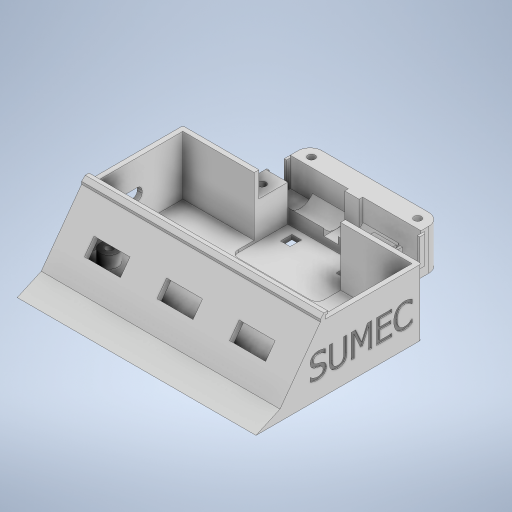
# Autodesk Inventor part: Sumec_telo_V4.1
Saved by Autodesk Inventor 2023 (Build 270158000, 158)
## iProperties
Created: 2023-03-18
Part Number: Sumec_telo_V4.1
Material: Všeobecné
Document SubType Name: Modeling
Designer: jaryj
Density: 1 g/cm^3
Appearance: Výchozí
Author: jaryj
Autodesk Inventor part; units mm, degrees
ref_plane "YZ Plane" through (0, 0, 0) normal (1, 0, 0) x (0, 1, 0)
ref_plane "XZ Plane" through (0, 0, 0) normal (0, 1, 0) x (-1, 0, 0)
ref_plane "XY Plane" through (0, 0, 0) normal (0, 0, 1) x (1, 0, 0)
sketch "Náčrt1" plane through (0, 0, 0) normal (0, 1, 0) x (-1, 0, 0)
  line L0 (0, 0) -> (49.75, 0)
  line L1 (49.75, 0) -> (49.75, -69)
  line L2 (49.75, -69) -> (18, -69)
  line L3 (18, -69) -> (18, -81)
  line L4 (18, -81) -> (27.25, -81)
  line L5 (27.25, -81) -> (27.25, -69)
  line L6 (27.25, -81) -> (27.25, -91.25)
  line L7 (27.25, -91.25) -> (27.25, -99.5)
  line L8 (27.25, -99.5) -> (0, -99.5)
  line L9 (0, -99.5) -> (0, -91.25)
  line L10 (0, -91.25) -> (27.25, -91.25)
  line L11 (0, -91.25) -> (0, -81)
  line L12 (0, -81) -> (18, -81)
  line L13 (0, -81) -> (0, 0)
  line L14 (18, -69) -> (18, -57.25)
  line L15 (18, -57.25) -> (0, -57.25)
  line L16 (47.75, -30) -> (47.75, -67)
  line L17 (47.75, -67) -> (18, -67)
  line L18 (0, -30) -> (47.75, -30)
  dimension "d0" = 49.75
  dimension "d1" = 69
  dimension "d2" = 12
  dimension "d3" = 10.25
  dimension "d4" = 8.25
  dimension "d5" = 27.25
  dimension "d6" = 18
  dimension "d9" = 2
  dimension "d13" = 30
  dimension "d18" = 2
  dimension "d190" = 9.75
  constraints: 38 end point, 12 perpendicular, 7 point on line, 1 horizontal, 1 vertical
  measures "d0" distance of L0.start L0.end
  measures "d1" distance of L0.end L1.end
  measures "d2" distance of L4.end L5.end
  measures "d3" distance of L4.end L6.end
  measures "d4" distance of L6.end L7.end
  measures "d5" distance of L7.end L8.end
  measures "d6" distance of L3.end L11.end
  measures "d9" distance between parallel lines of L17 L2
  measures "d13" distance between parallel lines of L0 L18
  measures "d18" distance between parallel lines of L1 L16
  measures "d190" distance between parallel lines of L17 L15
extrude "Vysunutí1" add sketch "Náčrt1" along normal blind 3 contours L18 L16 L17 L14 L15 L13
extrude "Vysunutí2" add sketch "Náčrt1" along normal blind 1.888 contours L15 L14 L3 L12 L13
extrude "Vysunutí3" add sketch "Náčrt1" along normal blind 27.5 contours L0 L1 L2 L14 L17 L16 L18 L13
extrude "Vysunutí4" add sketch "Náčrt1" along normal blind 17 contours L5 L4 L3 L2 | L10 L7 L8 L9
extrude "Vysunutí15" add sketch "Náčrt1" along normal blind 5 contours L12 L4 L6 L10 L11
sketch "Náčrt2" plane through (-49.75, 0, -69) normal (-1, 0, 0) x (0, 0, 1)
  line L0 (69, 0) -> (69, 27.5) projected
  line L1 (69, 0) -> (59, 4.5)
  line L2 (0, 0) -> (69, 0) projected
  line L3 (42.1707, 27.5) -> (59, 4.5)
  line L4 (69, 27.5) -> (0, 27.5) projected
  line L5 (69, 0) -> (69, 27.5) projected
  line L6 (69, 0) -> (69, 27.5)
  line L7 (69, 27.5) -> (42.1707, 27.5)
  point P0 (39, 27.5)
  point P1 (45.8293, 22.5)
  dimension "d24" = 4.5
  dimension "d25" = 10
  dimension "d235" = 53.807
  constraints: 8 end point, 1 collinear, 1 perpendicular, 1 point on line
  measures "d24" distance from line of L2 L1.end
  measures "d25" horizontal distance of L0.start L1.end
  measures "d235" angle of L2 L3
extrude "Vysunutí6" cut sketch "Náčrt2" against normal up to surface (49.75 mm away)
sketch "Náčrt3" plane through (0, 3, -30) normal (0, 0, -1) x (-1, 0, 0)
  line L0 (22.75, 15.167) -> (37.75, 15.167)
  line L1 (37.75, 15.167) -> (37.75, 0)
  line L2 (37.75, 0) -> (22.75, 0)
  line L3 (22.75, 0) -> (22.75, 15.167)
  line L4 (0, 15.167) -> (7.5, 15.167)
  line L5 (7.5, 15.167) -> (7.5, 0)
  line L6 (7.5, 0) -> (0, 0)
  line L7 (0, 0) -> (0, 15.167)
  line L8 (49.75, -3) -> (0, -3) projected
  dimension "d30" = 15
  dimension "d31" = 7.5
  dimension "d32" = 15.167
  dimension "d33" = 3
  dimension "d34" = 15.25
  constraints: 16 end point, 4 perpendicular, 4 point on line, 1 horizontal, 1 vertical alignment
  measures "d30" distance of L0.start L0.end
  measures "d31" distance of L4.start L4.end
  measures "d32" distance of L0.end L1.end
  measures "d33" distance between parallel lines of L8 L6
  measures "d34" distance between parallel lines of L3 L5
extrude "Vysunutí7" cut sketch "Náčrt3" against normal blind 14
sketch "Náčrt7" plane through (-47.75, 3, -67) normal (1, 0, 0) x (0, 0, -1)
  line L0 (-37, 0) -> (-50, 0)
  line L1 (-37, 0) -> (-51, 0) projected
  line L2 (-50, 0) -> (-50, 6.833)
  line L3 (-40.1707, 24.5) -> (2, 24.5) projected
  line L4 (2, -3) -> (-67, -3) projected
  line L5 (-40.1707, 24.5) -> (-46.9998, 15.167) projected
  line L6 (-37, 15.167) -> (-37, 24.5) projected
  line L7 (-37, 24.5) -> (-37, 0)
  line L8 (-37, 24.5) -> (-40.1707, 24.5) projected
  line L9 (-37.073, 24.5) -> (-37, 24.5)
  line L10 (-50, 6.833) -> (-37.073, 24.5)
  point P0 (-37, 15.167)
  dimension "d45" = 13
  dimension "d261" = 2.5
  constraints: 10 end point, 3 collinear, 2 perpendicular, 1 point on line
  measures "d45" distance of L0.start L0.end
  measures "d261" distance between parallel lines of L10 L5
extrude "Vysunutí9" cut sketch "Náčrt7" along normal through all
sketch "Náčrt13" plane through (0, 17, 0) normal (0, 1, 0) x (1, 0, 0)
  line L0 (-27.25, 81) -> (-18, 81) projected
  line L1 (-27.25, 69) -> (-27.25, 81) projected
  point P0 (0, 0)
  point P1 (-22.625, 75)
  dimension "d84" = 6
  dimension "d85" = 4.625
  measures "d84" distance from line of L0 point (-22.625, 75)
  measures "d85" distance from line of L1 point (-22.625, 75)
hole "Díra2" at (-22.625, 17, -75) direction (0, -1, 0) diameter 3 depth 6
sketch "Náčrt14" plane through (0, 17, 0) normal (0, 1, 0) x (1, 0, 0)
  line L0 (-27.25, 91.25) -> (-27.25, 99.5) projected
  line L1 (-27.25, 99.5) -> (0, 99.5) projected
  point P0 (0, 0)
  point P1 (-22.125, 95)
  dimension "d93" = 5.125
  dimension "d101" = 4.5
  measures "d93" distance from line of L0 point (-22.125, 95)
  measures "d101" distance from line of L1 point (-22.125, 95)
hole "Díra3" at (-22.125, 17, -95) direction (0, -1, 0) diameter 3 depth 6
fillet "Zaoblení1" radius 3 1 edges at (-18, 2.444, -57.25)
fillet "Zaoblení2" radius 1 1 edges at (-49.75, 13.75, -69)
fillet "Zaoblení3" radius 5 1 edges at (-27.25, 8.5, -99.5)
sketch "Náčrt24" plane through (-18, 3, -67) normal (1, 0, 0) x (0, 0, -1)
  line L0 (24.25, 2) -> (24.25, 14) projected
  line L1 (14, 2) -> (24.25, 2) projected
  line L2 (14, 2) -> (14, 14) projected
  line L3 (24.25, 2) -> (14, 2) projected
  line L4 (24.25, 4.88) -> (24.25, 2)
  line L5 (24.25, 2) -> (14, 2)
  line L6 (14, 2) -> (14, 4.88)
  arc A0 (14, 4.88) -> (24.25, 4.88) centre (19.125, 8) ccw
  point P0 (-67, -3)
  point P1 (19.125, 2)
  dimension "d200" = 6
  constraints: 6 end point, 2 perpendicular, 2 point on circle, 2 point on line, 1 centre point, 1 horizontal alignment, 1 tangent
  measures "d200" radius of A0
extrude "Vysunutí22" add sketch "Náčrt24" along normal blind 15
sketch "Náčrt21" plane through (-27.25, 0, -69) normal (-1, 0, 0) x (0, 0, 1)
  line L0 (-20.75, 16) -> (-23.75, 16)
  line L1 (-30.5, 17) -> (-22.25, 17) projected
  line L2 (-23.75, 3.5) -> (-10.5, 3.5)
  line L3 (-10.5, 3.5) -> (-10.5, 16)
  line L4 (-10.5, 16) -> (-13.5, 16)
  line L5 (-13.5, 16) -> (-13.5, 6.5)
  line L6 (-13.5, 6.5) -> (-20.75, 6.5)
  line L7 (-20.75, 6.5) -> (-20.75, 16)
  line L8 (-23.75, 16) -> (-23.75, 3.5)
  line L9 (-22.25, 5) -> (-22.25, 17) projected
  line L10 (-12, 5) -> (-22.25, 5) projected
  line L11 (-12, 5) -> (-12, 17) projected
  line L12 (0, 17) -> (-12, 17) projected
  point P0 (69, 0)
  dimension "d172" = 1.5
  dimension "d173" = 1.5
  dimension "d174" = 1.5
  dimension "d175" = 1.5
  dimension "d176" = 1.5
  dimension "d177" = 1.5
  dimension "d180" = 1
  constraints: 12 end point, 3 perpendicular, 1 horizontal, 1 parallel, 1 vertical, 8 other
  measures "d172" distance between parallel lines of L7 L9
  measures "d173" distance between parallel lines of L6 L10
  measures "d174" distance between parallel lines of L5 L11
  measures "d175" distance between parallel lines of L11 L3
  measures "d176" distance between parallel lines of L2 L10
  measures "d177" distance between parallel lines of L8 L9
extrude "Vysunutí19" add sketch "Náčrt21" along normal blind 1
chamfer "Zkosení1" distance 1 angle 45 3 edges at (-28.25, 9.75, -92.75) (-28.25, 3.5, -86.125) (-28.25, 9.75, -79.5)
mirror "Zrcadlit1" about plane through (0, 0, -99.5) normal (1, 0, 0)
sketch "Náčrt30" plane through (-49.75, 0, -68) normal (-1, 0, 0) x (0, 0, 1)
  line L0 (58, 4.5) -> (41.1707, 27.5) projected
  line L1 (41.1707, 27.5) -> (41.1707, 30)
  line L2 (41.1707, 30) -> (38.073, 30)
  line L3 (38.073, 30) -> (38.073, 29)
  line L4 (38.073, 29) -> (39.073, 29)
  line L5 (39.073, 29) -> (39.073, 27.5)
  line L6 (41.1707, 27.5) -> (0, 27.5) projected
  line L7 (39.073, 27.5) -> (41.1707, 27.5)
  line L8 (38.073, 27.5) -> (51, 9.833) projected
  point P0 (68, 0)
  point P1 (39.073, 27.5)
  dimension "d236" = 1.5
  dimension "d237" = 1
  dimension "d263" = 1
  constraints: 12 end point, 4 perpendicular, 1 collinear, 1 horizontal, 1 vertical alignment
  measures "d236" distance of L4.end L5.end
  measures "d237" distance of L3.end L4.end
  measures "d263" distance of L2.end L3.end
sketch "Náčrt16" plane through (0, 1.888, 0) normal (0, 1, 0) x (1, 0, 0)
  line L0 (-9.4, 73.375) -> (-13.4, 73.375)
  line L1 (-13.4, 73.375) -> (-13.4, 78.125)
  line L2 (-13.4, 78.125) -> (-9.4, 78.125)
  line L3 (-9.4, 78.125) -> (-9.4, 73.375)
  line L4 (-18, 81) -> (-18, 69) projected
  line L5 (13.75, 73.375) -> (9.75, 73.375)
  line L6 (9.75, 73.375) -> (9.75, 78.125)
  line L7 (9.75, 78.125) -> (13.75, 78.125)
  line L8 (13.75, 78.125) -> (13.75, 73.375)
  line L9 (18, 81) -> (18, 69) projected
  line L10 (-18, 81) -> (18, 81) projected
  point P0 (0, 0)
  dimension "d128" = 4
  dimension "d129" = 4.75
  dimension "d130" = 4.6
  dimension "d134" = 4.25
  dimension "d192" = 2.875
  constraints: 16 end point, 4 parallel, 2 equal length, 2 perpendicular, 1 horizontal, 1 horizontal alignment
  measures "d128" distance of L0.start L0.end
  measures "d129" distance of L2.end L0.start
  measures "d130" distance between parallel lines of L4 L1
  measures "d134" distance between parallel lines of L9 L8
  measures "d192" distance between parallel lines of L10 L2
extrude "Vysunutí16" cut sketch "Náčrt16" against normal through all
sketch "Náčrt17" plane through (0, 3, 0) normal (0, 1, 0) x (1, 0, 0)
  line L0 (-47.75, 17) -> (-37.75, 17) projected
  line L1 (-47.75, 17) -> (-47.75, 67) projected
  line L2 (47.75, 17) -> (37.75, 17) projected
  line L3 (47.75, 17) -> (47.75, 67) projected
  line L4 (-39.4, 19.625) -> (-43.4, 19.625)
  line L5 (-43.4, 19.625) -> (-43.4, 24.375)
  line L6 (-43.4, 24.375) -> (-39.4, 24.375)
  line L7 (-39.4, 24.375) -> (-39.4, 19.625)
  line L8 (42.75, 19.625) -> (38.75, 19.625)
  line L9 (38.75, 19.625) -> (38.75, 24.375)
  line L10 (38.75, 24.375) -> (42.75, 24.375)
  line L11 (42.75, 24.375) -> (42.75, 19.625)
  point P0 (0, 0)
  point P1 (-48, 67)
  point P2 (48, 67)
  point P3 (-41.4, 19.625)
  point P4 (40.75, 19.625)
  point P5 (-47.75, 67)
  dimension "d137" = 4
  dimension "d138" = 4.75
  dimension "d139" = 4.35
  dimension "d143" = 2.625
  dimension "d144" = 5
  dimension "d146" = 2.625
  constraints: 16 end point, 4 parallel, 2 equal length, 2 horizontal, 2 midpoint, 2 perpendicular, 2 other
  measures "d137" distance of L4.start L4.end
  measures "d138" distance of L6.end L4.start
  measures "d143" distance between parallel lines of L0 L4
  measures "d146" distance from line of L2 point (40.75, 19.625)
extrude "Vysunutí17" cut sketch "Náčrt17" against normal through all
sketch "Náčrt18" plane through (0, 3, 0) normal (0, 1, 0) x (1, 0, 0)
  circle A0 centre (39.25, 59) radius 3.75
  circle A1 centre (-40.5, 29) radius 3.75
  line L0 (18, 67) -> (47.75, 67) projected
  line L1 (-47.75, 17) -> (-37.75, 17) projected
  line L2 (-47.75, 17) -> (-47.75, 67) projected
  line L3 (47.75, 17) -> (47.75, 67) projected
  point P0 (0, 0)
  point P1 (42.5, 67)
  point P2 (-48, 67)
  point P3 (-47.75, 67)
  dimension "d149" = 7.5
  dimension "d150" = 8
  dimension "d152" = 12
  dimension "d153" = 7.25
  dimension "d262" = 8.5
  constraints: 2 centre point, 1 equal radius, 1 other
  measures "d149" diameter of A0
  measures "d150" distance from line of A0.centre L0
  measures "d152" distance from line of L1 A1.centre
  measures "d262" distance from line of L3 A0.centre
extrude "Vysunutí18" add sketch "Náčrt18" along normal blind 5
sketch "Náčrt19" plane through (39.25, 8, -59) normal (0, 1, 0) x (1, 0, 0)
  circle A0 centre (0, 0) radius 3.75 projected
  point P0 (-39.25, -59)
  constraints: 1 coincident
hole "Díra4" at (39.25, 8, -59) direction (0, -1, 0) diameter 3 depth 6
sketch "Náčrt20" plane through (-40.5, 8, -29) normal (0, 1, 0) x (1, 0, 0)
  circle A0 centre (0, 0) radius 3.75 projected
  point P0 (40.5, -29)
  point P1 (-3.6436, 0.8871)
  point P2 (3.75, 0)
  constraints: 1 coincident
hole "Díra5" at (-40.5, 8, -29) direction (0, -1, 0) diameter 3 depth 6
sketch "Náčrt25" plane through (-18, 7.88, -91.25) normal (0, 0, 1) x (1, 0, 0)
  line L0 (40.25, 9.12) -> (-4.25, 9.12) projected
  line L1 (15, 9.12) -> (21, 9.12)
  line L2 (21, 9.12) -> (21, -2.88)
  line L3 (21, -2.88) -> (15, -2.88)
  line L4 (15, -2.88) -> (15, 9.12)
  line L5 (15, -2.88) -> (15, 0) projected
  line L6 (21, -2.88) -> (21, 0) projected
  point P0 (18, -7.88)
  dimension "d203" = 12
  dimension "d204" = 6
  constraints: 8 end point, 2 parallel, 1 coincident, 1 horizontal, 1 perpendicular, 1 point on line
  measures "d203" distance of L3.end L1.start
  measures "d204" distance between parallel lines of L2 L4
extrude "Vysunutí23" add sketch "Náčrt25" along normal blind 1.5
sketch "Náčrt26" plane through (-49.75, 0, -68) normal (-1, 0, 0) x (0, 0, 1)
  line L0 (20, 11.7) -> (27, 11.7)
  line L1 (27, 16.7) -> (20, 16.7)
  line L2 (18, 14.7) -> (18, 13.7)
  line L3 (29, 14.7) -> (29, 13.7)
  line L4 (0, 0) -> (68, 0) projected
  line L5 (0, 0) -> (0, 27.5) projected
  arc A0 (20, 16.7) -> (18, 14.7) centre (20, 14.7) ccw
  arc A1 (18, 13.7) -> (20, 11.7) centre (20, 13.7) ccw
  arc A2 (29, 14.7) -> (27, 16.7) centre (27, 14.7) ccw
  arc A3 (27, 11.7) -> (29, 13.7) centre (27, 13.7) ccw
  dimension "d207" = 11.7
  dimension "d208" = 5
  dimension "d209" = 11
  dimension "d210" = 18
  dimension "d211" = 2
  constraints: 8 end point, 8 point on circle, 8 tangent, 4 centre point, 3 equal radius, 1 horizontal, 1 parallel, 1 vertical
  measures "d207" distance between parallel lines of L4 L0
  measures "d208" distance between parallel lines of L0 L1
  measures "d209" distance between parallel lines of L3 L2
  measures "d210" distance between parallel lines of L5 L2
  measures "d211" radius of A0
extrude "Vysunutí24" cut sketch "Náčrt26" against normal up to surface (2 mm away)
sketch "Náčrt28" plane through (49.75, 0, 0) normal (1, 0, 0) x (0, 0, -1)
  line L0 (22, 17.5) -> (66, 17.5) construction
  line L1 (66, 17.5) -> (66, 7) construction
  line L2 (66, 7) -> (22, 7) construction
  line L3 (22, 7) -> (22, 17.5) construction
  line L4 (26.8293, 27.5) -> (68, 27.5) projected
  line L5 (68, 0) -> (68, 27.5) projected
  line L6 (69, 27.5) -> (69, 0) projected
  spline S0 degree 2 poles (25.8006, 7.1434) (24.7147, 7.1434) (23.1912, 7.5972) (22.5186, 7.9214) knots 0 0 0 1 2 2 2
  line L7 (22.5186, 7.9214) -> (22.5186, 9.5908)
  line L8 (22.5186, 9.5908) -> (22.6159, 9.5908)
  spline S1 degree 2 poles (22.6159, 9.5908) (23.2723, 8.9749) (24.9335, 8.2942) (25.7034, 8.2942) knots 0 0 0 1 2 2 2
  spline S2 degree 2 poles (25.7034, 8.2942) (26.8055, 8.2942) (27.9319, 9.2099) (27.9319, 9.9635) knots 0 0 0 1 2 2 2
  spline S3 degree 2 poles (27.9319, 9.9635) (27.9319, 10.5632) (27.3404, 11.3088) (26.7002, 11.4951) knots 0 0 0 1 2 2 2
  spline S4 degree 2 poles (26.7002, 11.4951) (26.2382, 11.6248) (25.4684, 11.8031) (24.893, 11.9489) knots 0 0 0 1 2 2 2
  spline S5 degree 2 poles (24.893, 11.9489) (24.3744, 12.0867) (23.5559, 12.5) (23.2399, 12.8323) knots 0 0 0 1 2 2 2
  spline S6 degree 2 poles (23.2399, 12.8323) (22.9319, 13.1645) (22.5916, 14.0559) (22.5916, 14.6394) knots 0 0 0 1 2 2 2
  spline S7 degree 2 poles (22.5916, 14.6394) (22.5916, 15.8549) (24.4878, 17.5) (25.9546, 17.5) knots 0 0 0 1 2 2 2
  spline S8 degree 2 poles (25.9546, 17.5) (26.7974, 17.5) (28.2885, 17.1677) (28.9287, 16.8517) knots 0 0 0 1 2 2 2
  line L9 (28.9287, 16.8517) -> (28.9287, 15.2634)
  line L10 (28.9287, 15.2634) -> (28.8314, 15.2634)
  spline S9 degree 2 poles (28.8314, 15.2634) (28.3533, 15.701) (26.8622, 16.3493) (26.0438, 16.3493) knots 0 0 0 1 2 2 2
  spline S10 degree 2 poles (26.0438, 16.3493) (25.1199, 16.3493) (23.9773, 15.4822) (23.9773, 14.7771) knots 0 0 0 1 2 2 2
  spline S11 degree 2 poles (23.9773, 14.7771) (23.9773, 14.1451) (24.6499, 13.3914) (25.282, 13.2212) knots 0 0 0 1 2 2 2
  spline S12 degree 2 poles (25.282, 13.2212) (25.7034, 13.1078) (26.9271, 12.816) (27.3323, 12.6945) knots 0 0 0 1 2 2 2
  spline S13 degree 2 poles (27.3323, 12.6945) (28.3614, 12.3784) (29.3177, 11.1062) (29.3177, 10.1742) knots 0 0 0 1 2 2 2
  spline S14 degree 2 poles (29.3177, 10.1742) (29.3177, 9.5827) (28.8395, 8.4481) (28.41, 8.0511) knots 0 0 0 1 2 2 2
  spline S15 degree 2 poles (28.41, 8.0511) (27.9319, 7.6135) (26.7164, 7.1434) (25.8006, 7.1434) knots 0 0 0 1 2 2 2
  spline S16 degree 2 poles (34.1637, 7.111) (33.2804, 7.111) (31.9676, 7.5729) (31.5057, 8.0348) knots 0 0 0 1 2 2 2
  spline S17 degree 2 poles (31.5057, 8.0348) (30.9789, 8.5535) (30.5494, 10.0122) (30.5494, 11.0818) knots 0 0 0 1 2 2 2
  line L11 (30.5494, 11.0818) -> (30.5494, 17.3217)
  line L12 (30.5494, 17.3217) -> (31.8784, 17.3217)
  line L13 (31.8784, 17.3217) -> (31.8784, 11.0818)
  spline S18 degree 2 poles (31.8784, 11.0818) (31.8784, 10.3849) (32.0567, 9.4449) (32.3079, 9.064) knots 0 0 0 1 2 2 2
  spline S19 degree 2 poles (32.3079, 9.064) (32.5754, 8.6588) (33.4992, 8.2455) (34.1637, 8.2455) knots 0 0 0 1 2 2 2
  spline S20 degree 2 poles (34.1637, 8.2455) (34.7877, 8.2455) (35.7601, 8.6588) (36.0276, 9.064) knots 0 0 0 1 2 2 2
  spline S21 degree 2 poles (36.0276, 9.064) (36.2788, 9.4449) (36.4571, 10.3768) (36.4571, 11.0494) knots 0 0 0 1 2 2 2
  line L14 (36.4571, 11.0494) -> (36.4571, 17.3217)
  line L15 (36.4571, 17.3217) -> (37.7861, 17.3217)
  line L16 (37.7861, 17.3217) -> (37.7861, 11.0818)
  spline S22 degree 2 poles (37.7861, 11.0818) (37.7861, 10.0365) (37.3647, 8.5454) (36.8298, 8.0348) knots 0 0 0 1 2 2 2
  spline S23 degree 2 poles (36.8298, 8.0348) (36.3517, 7.5648) (35.0875, 7.111) (34.1637, 7.111) knots 0 0 0 1 2 2 2
  line L17 (48.2642, 7.3217) -> (46.9352, 7.3217)
  line L18 (46.9352, 7.3217) -> (46.9352, 15.936)
  line L19 (46.9352, 15.936) -> (44.3258, 10.077)
  line L20 (44.3258, 10.077) -> (43.5154, 10.077)
  line L21 (43.5154, 10.077) -> (40.9303, 15.936)
  line L22 (40.9303, 15.936) -> (40.9303, 7.3217)
  line L23 (40.9303, 7.3217) -> (39.6904, 7.3217)
  line L24 (39.6904, 7.3217) -> (39.6904, 17.3217)
  line L25 (39.6904, 17.3217) -> (41.5057, 17.3217)
  line L26 (41.5057, 17.3217) -> (44.0016, 11.7545)
  line L27 (44.0016, 11.7545) -> (46.4165, 17.3217)
  line L28 (46.4165, 17.3217) -> (48.2642, 17.3217)
  line L29 (48.2642, 17.3217) -> (48.2642, 7.3217)
  line L30 (50.2901, 7.3217) -> (50.2901, 17.3217)
  line L31 (50.2901, 17.3217) -> (56.5462, 17.3217)
  line L32 (56.5462, 17.3217) -> (56.5462, 16.1386)
  line L33 (56.5462, 16.1386) -> (51.6191, 16.1386)
  line L34 (51.6191, 16.1386) -> (51.6191, 13.3995)
  line L35 (51.6191, 13.3995) -> (56.2139, 13.3995)
  line L36 (56.2139, 13.3995) -> (56.2139, 12.2164)
  line L37 (56.2139, 12.2164) -> (51.6191, 12.2164)
  line L38 (51.6191, 12.2164) -> (51.6191, 8.5049)
  line L39 (51.6191, 8.5049) -> (56.5462, 8.5049)
  line L40 (56.5462, 8.5049) -> (56.5462, 7.3217)
  line L41 (56.5462, 7.3217) -> (50.2901, 7.3217)
  spline S24 degree 2 poles (61.9109, 7.1434) (60.9384, 7.1434) (59.2934, 7.7998) (58.6937, 8.4562) knots 0 0 0 1 2 2 2
  spline S25 degree 2 poles (58.6937, 8.4562) (58.094, 9.1045) (57.4376, 11.0494) (57.4376, 12.3136) knots 0 0 0 1 2 2 2
  spline S26 degree 2 poles (57.4376, 12.3136) (57.4376, 13.5697) (58.0778, 15.4335) (58.6856, 16.1224) knots 0 0 0 1 2 2 2
  spline S27 degree 2 poles (58.6856, 16.1224) (59.2853, 16.795) (60.9222, 17.5) (61.9352, 17.5) knots 0 0 0 1 2 2 2
  spline S28 degree 2 poles (61.9352, 17.5) (62.4376, 17.5) (63.3209, 17.3541) (63.6937, 17.2407) knots 0 0 0 1 2 2 2
  spline S29 degree 2 poles (63.6937, 17.2407) (64.0178, 17.1353) (64.6904, 16.8355) (65.0227, 16.6572) knots 0 0 0 1 2 2 2
  line L42 (65.0227, 16.6572) -> (65.0227, 15.0527)
  line L43 (65.0227, 15.0527) -> (64.9173, 15.0527)
  spline S30 degree 2 poles (64.9173, 15.0527) (64.7391, 15.2147) (64.188, 15.6686) (63.7909, 15.8874) knots 0 0 0 1 2 2 2
  spline S31 degree 2 poles (63.7909, 15.8874) (63.41, 16.0981) (62.5105, 16.3655) (61.9271, 16.3655) knots 0 0 0 1 2 2 2
  spline S32 degree 2 poles (61.9271, 16.3655) (61.2869, 16.3655) (60.1442, 15.8387) (59.7147, 15.3363) knots 0 0 0 1 2 2 2
  spline S33 degree 2 poles (59.7147, 15.3363) (59.2934, 14.8258) (58.8233, 13.278) (58.8233, 12.3136) knots 0 0 0 1 2 2 2
  spline S34 degree 2 poles (58.8233, 12.3136) (58.8233, 11.2844) (59.3177, 9.8015) (59.7472, 9.2909) knots 0 0 0 1 2 2 2
  spline S35 degree 2 poles (59.7472, 9.2909) (60.1686, 8.7966) (61.295, 8.2942) (61.9271, 8.2942) knots 0 0 0 1 2 2 2
  spline S36 degree 2 poles (61.9271, 8.2942) (62.5024, 8.2942) (63.483, 8.5778) (63.8639, 8.7885) knots 0 0 0 1 2 2 2
  spline S37 degree 2 poles (63.8639, 8.7885) (64.2285, 8.9992) (64.7715, 9.4368) (64.9254, 9.5908) knots 0 0 0 1 2 2 2
  line L44 (64.9254, 9.5908) -> (65.0227, 9.5908)
  line L45 (65.0227, 9.5908) -> (65.0227, 8.0024)
  spline S38 degree 2 poles (65.0227, 8.0024) (64.6904, 7.8485) (64.107, 7.5648) (63.6937, 7.4352) knots 0 0 0 1 2 2 2
  spline S39 degree 2 poles (63.6937, 7.4352) (63.2561, 7.2893) (62.5105, 7.1434) (61.9109, 7.1434) knots 0 0 0 1 2 2 2
  point P0 (0, 0)
  point P1 (25, 22.5)
  point P2 (0, 27.5)
  dimension "d229" = 10
  dimension "d231" = 44
  dimension "d232" = 10.5
  dimension "d264" = 3
  constraints: 3 other
  measures "d231" distance of L0.start L0.end
  measures "d232" distance of L2.end L0.start
  measures "d264" distance between parallel lines of L6 L1
extrude "Vysunutí26" cut sketch "Náčrt28" against normal blind 0.4
sketch "Náčrt29" plane through (-49.75, 0, -68) normal (-1, 0, 0) x (0, 0, 1)
  line L0 (2, 17.5) -> (46, 17.5) construction
  line L1 (46, 17.5) -> (46, 7) construction
  line L2 (46, 7) -> (2, 7) construction
  line L3 (2, 7) -> (2, 17.5) construction
  line L4 (41.1707, 27.5) -> (0, 27.5) projected
  line L5 (-1, 27.5) -> (-1, 0) projected
  spline S0 degree 2 poles (5.8006, 7.1434) (4.7147, 7.1434) (3.1912, 7.5972) (2.5186, 7.9214) knots 0 0 0 1 2 2 2
  line L6 (2.5186, 7.9214) -> (2.5186, 9.5908)
  line L7 (2.5186, 9.5908) -> (2.6159, 9.5908)
  spline S1 degree 2 poles (2.6159, 9.5908) (3.2723, 8.9749) (4.9335, 8.2942) (5.7034, 8.2942) knots 0 0 0 1 2 2 2
  spline S2 degree 2 poles (5.7034, 8.2942) (6.8055, 8.2942) (7.9319, 9.2099) (7.9319, 9.9635) knots 0 0 0 1 2 2 2
  spline S3 degree 2 poles (7.9319, 9.9635) (7.9319, 10.5632) (7.3404, 11.3088) (6.7002, 11.4951) knots 0 0 0 1 2 2 2
  spline S4 degree 2 poles (6.7002, 11.4951) (6.2382, 11.6248) (5.4684, 11.8031) (4.893, 11.9489) knots 0 0 0 1 2 2 2
  spline S5 degree 2 poles (4.893, 11.9489) (4.3744, 12.0867) (3.5559, 12.5) (3.2399, 12.8323) knots 0 0 0 1 2 2 2
  spline S6 degree 2 poles (3.2399, 12.8323) (2.9319, 13.1645) (2.5916, 14.0559) (2.5916, 14.6394) knots 0 0 0 1 2 2 2
  spline S7 degree 2 poles (2.5916, 14.6394) (2.5916, 15.8549) (4.4878, 17.5) (5.9546, 17.5) knots 0 0 0 1 2 2 2
  spline S8 degree 2 poles (5.9546, 17.5) (6.7974, 17.5) (8.2885, 17.1677) (8.9287, 16.8517) knots 0 0 0 1 2 2 2
  line L8 (8.9287, 16.8517) -> (8.9287, 15.2634)
  line L9 (8.9287, 15.2634) -> (8.8314, 15.2634)
  spline S9 degree 2 poles (8.8314, 15.2634) (8.3533, 15.701) (6.8622, 16.3493) (6.0438, 16.3493) knots 0 0 0 1 2 2 2
  spline S10 degree 2 poles (6.0438, 16.3493) (5.1199, 16.3493) (3.9773, 15.4822) (3.9773, 14.7771) knots 0 0 0 1 2 2 2
  spline S11 degree 2 poles (3.9773, 14.7771) (3.9773, 14.1451) (4.6499, 13.3914) (5.282, 13.2212) knots 0 0 0 1 2 2 2
  spline S12 degree 2 poles (5.282, 13.2212) (5.7034, 13.1078) (6.9271, 12.816) (7.3323, 12.6945) knots 0 0 0 1 2 2 2
  spline S13 degree 2 poles (7.3323, 12.6945) (8.3614, 12.3784) (9.3177, 11.1062) (9.3177, 10.1742) knots 0 0 0 1 2 2 2
  spline S14 degree 2 poles (9.3177, 10.1742) (9.3177, 9.5827) (8.8395, 8.4481) (8.41, 8.0511) knots 0 0 0 1 2 2 2
  spline S15 degree 2 poles (8.41, 8.0511) (7.9319, 7.6135) (6.7164, 7.1434) (5.8006, 7.1434) knots 0 0 0 1 2 2 2
  spline S16 degree 2 poles (14.1637, 7.111) (13.2804, 7.111) (11.9676, 7.5729) (11.5057, 8.0348) knots 0 0 0 1 2 2 2
  spline S17 degree 2 poles (11.5057, 8.0348) (10.9789, 8.5535) (10.5494, 10.0122) (10.5494, 11.0818) knots 0 0 0 1 2 2 2
  line L10 (10.5494, 11.0818) -> (10.5494, 17.3217)
  line L11 (10.5494, 17.3217) -> (11.8784, 17.3217)
  line L12 (11.8784, 17.3217) -> (11.8784, 11.0818)
  spline S18 degree 2 poles (11.8784, 11.0818) (11.8784, 10.3849) (12.0567, 9.4449) (12.3079, 9.064) knots 0 0 0 1 2 2 2
  spline S19 degree 2 poles (12.3079, 9.064) (12.5754, 8.6588) (13.4992, 8.2455) (14.1637, 8.2455) knots 0 0 0 1 2 2 2
  spline S20 degree 2 poles (14.1637, 8.2455) (14.7877, 8.2455) (15.7601, 8.6588) (16.0276, 9.064) knots 0 0 0 1 2 2 2
  spline S21 degree 2 poles (16.0276, 9.064) (16.2788, 9.4449) (16.4571, 10.3768) (16.4571, 11.0494) knots 0 0 0 1 2 2 2
  line L13 (16.4571, 11.0494) -> (16.4571, 17.3217)
  line L14 (16.4571, 17.3217) -> (17.7861, 17.3217)
  line L15 (17.7861, 17.3217) -> (17.7861, 11.0818)
  spline S22 degree 2 poles (17.7861, 11.0818) (17.7861, 10.0365) (17.3647, 8.5454) (16.8298, 8.0348) knots 0 0 0 1 2 2 2
  spline S23 degree 2 poles (16.8298, 8.0348) (16.3517, 7.5648) (15.0875, 7.111) (14.1637, 7.111) knots 0 0 0 1 2 2 2
  line L16 (28.2642, 7.3217) -> (26.9352, 7.3217)
  line L17 (26.9352, 7.3217) -> (26.9352, 15.936)
  line L18 (26.9352, 15.936) -> (24.3258, 10.077)
  line L19 (24.3258, 10.077) -> (23.5154, 10.077)
  line L20 (23.5154, 10.077) -> (20.9303, 15.936)
  line L21 (20.9303, 15.936) -> (20.9303, 7.3217)
  line L22 (20.9303, 7.3217) -> (19.6904, 7.3217)
  line L23 (19.6904, 7.3217) -> (19.6904, 17.3217)
  line L24 (19.6904, 17.3217) -> (21.5057, 17.3217)
  line L25 (21.5057, 17.3217) -> (24.0016, 11.7545)
  line L26 (24.0016, 11.7545) -> (26.4165, 17.3217)
  line L27 (26.4165, 17.3217) -> (28.2642, 17.3217)
  line L28 (28.2642, 17.3217) -> (28.2642, 7.3217)
  line L29 (30.2901, 7.3217) -> (30.2901, 17.3217)
  line L30 (30.2901, 17.3217) -> (36.5462, 17.3217)
  line L31 (36.5462, 17.3217) -> (36.5462, 16.1386)
  line L32 (36.5462, 16.1386) -> (31.6191, 16.1386)
  line L33 (31.6191, 16.1386) -> (31.6191, 13.3995)
  line L34 (31.6191, 13.3995) -> (36.2139, 13.3995)
  line L35 (36.2139, 13.3995) -> (36.2139, 12.2164)
  line L36 (36.2139, 12.2164) -> (31.6191, 12.2164)
  line L37 (31.6191, 12.2164) -> (31.6191, 8.5049)
  line L38 (31.6191, 8.5049) -> (36.5462, 8.5049)
  line L39 (36.5462, 8.5049) -> (36.5462, 7.3217)
  line L40 (36.5462, 7.3217) -> (30.2901, 7.3217)
  spline S24 degree 2 poles (41.9109, 7.1434) (40.9384, 7.1434) (39.2934, 7.7998) (38.6937, 8.4562) knots 0 0 0 1 2 2 2
  spline S25 degree 2 poles (38.6937, 8.4562) (38.094, 9.1045) (37.4376, 11.0494) (37.4376, 12.3136) knots 0 0 0 1 2 2 2
  spline S26 degree 2 poles (37.4376, 12.3136) (37.4376, 13.5697) (38.0778, 15.4335) (38.6856, 16.1224) knots 0 0 0 1 2 2 2
  spline S27 degree 2 poles (38.6856, 16.1224) (39.2853, 16.795) (40.9222, 17.5) (41.9352, 17.5) knots 0 0 0 1 2 2 2
  spline S28 degree 2 poles (41.9352, 17.5) (42.4376, 17.5) (43.3209, 17.3541) (43.6937, 17.2407) knots 0 0 0 1 2 2 2
  spline S29 degree 2 poles (43.6937, 17.2407) (44.0178, 17.1353) (44.6904, 16.8355) (45.0227, 16.6572) knots 0 0 0 1 2 2 2
  line L41 (45.0227, 16.6572) -> (45.0227, 15.0527)
  line L42 (45.0227, 15.0527) -> (44.9173, 15.0527)
  spline S30 degree 2 poles (44.9173, 15.0527) (44.7391, 15.2147) (44.188, 15.6686) (43.7909, 15.8874) knots 0 0 0 1 2 2 2
  spline S31 degree 2 poles (43.7909, 15.8874) (43.41, 16.0981) (42.5105, 16.3655) (41.9271, 16.3655) knots 0 0 0 1 2 2 2
  spline S32 degree 2 poles (41.9271, 16.3655) (41.2869, 16.3655) (40.1442, 15.8387) (39.7147, 15.3363) knots 0 0 0 1 2 2 2
  spline S33 degree 2 poles (39.7147, 15.3363) (39.2934, 14.8258) (38.8233, 13.278) (38.8233, 12.3136) knots 0 0 0 1 2 2 2
  spline S34 degree 2 poles (38.8233, 12.3136) (38.8233, 11.2844) (39.3177, 9.8015) (39.7472, 9.2909) knots 0 0 0 1 2 2 2
  spline S35 degree 2 poles (39.7472, 9.2909) (40.1686, 8.7966) (41.295, 8.2942) (41.9271, 8.2942) knots 0 0 0 1 2 2 2
  spline S36 degree 2 poles (41.9271, 8.2942) (42.5024, 8.2942) (43.483, 8.5778) (43.8639, 8.7885) knots 0 0 0 1 2 2 2
  spline S37 degree 2 poles (43.8639, 8.7885) (44.2285, 8.9992) (44.7715, 9.4368) (44.9254, 9.5908) knots 0 0 0 1 2 2 2
  line L43 (44.9254, 9.5908) -> (45.0227, 9.5908)
  line L44 (45.0227, 9.5908) -> (45.0227, 8.0024)
  spline S38 degree 2 poles (45.0227, 8.0024) (44.6904, 7.8485) (44.107, 7.5648) (43.6937, 7.4352) knots 0 0 0 1 2 2 2
  spline S39 degree 2 poles (43.6937, 7.4352) (43.2561, 7.2893) (42.5105, 7.1434) (41.9109, 7.1434) knots 0 0 0 1 2 2 2
  point P0 (68, 0)
  point P1 (43, 22.5)
  point P2 (68, 27.5)
  dimension "d225" = 10
  dimension "d226" = 3
  dimension "d233" = 44
  dimension "d234" = 10.5
  constraints: 3 other
  measures "d226" distance between parallel lines of L5 L3
  measures "d233" distance of L0.start L0.end
  measures "d234" distance of L0.end L1.end
extrude "Vysunutí27" cut sketch "Náčrt29" against normal blind 0.4
extrude "Vysunutí28" add sketch "Náčrt30" against normal up to surface (99.5 mm away)
chamfer "Zkosení2" distance 1.5 angle 45 1 edges at (0, 30, -26.8293)
